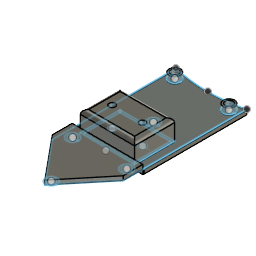
extension (Autodesk Fusion 360 design; units mm, degrees)
part number: 2025-12-24-19-58-26-619
Autodesk Fusion 360 part; units mm, degrees
sketch "Sketch1" plane through (0, 0, 0) normal (0, 0, 1) x (1, 0, 0)
  line L0 (-17.024, 124.2448) -> (-17.024, 75)
  line L1 (17.0001, 124.2453) -> (17.0001, 75)
  circle A0 centre (-13.0088, 119.745) radius 1.85
  circle A1 centre (-13.0088, 119.745) radius 2.75
  circle A2 centre (12.9912, 119.745) radius 1.85
  circle A3 centre (12.9912, 119.745) radius 2.75
  circle A4 centre (-7.3385, 84.0106) radius 1.5
  circle A5 centre (0, 96.5) radius 1.85
  circle A6 centre (0, 96.5) radius 2.75
  spline S0 degree 5 poles (-17.024, 124.2448) (-16.3297, 124.0957) (-14.9423, 123.8106) (-12.8649, 123.4218) (-10.1022, 122.9825) (-6.662, 122.574) (-3.236, 122.3191) (0.1747, 122.2305) (3.5692, 122.3158) (6.9481, 122.5687) (10.3127, 122.977) (12.9938, 123.4177) (14.9991, 123.8085) (16.3335, 124.0953) (17.0001, 124.2453) knots 0 0 0 0 0 0 0.1 0.2 0.3 0.4 0.5 0.6 0.7 0.8 0.9 1 1 1 1 1 1
  line L2 (13.0005, 74.4499) -> (-13.1768, 74.5708)
  line L3 (-13.089, 93.5708) -> (12.9107, 93.6922)
  line L4 (-13.089, 93.5708) -> (-13.1768, 74.5708)
  line L5 (13.0005, 74.4499) -> (12.9107, 93.6922)
  line L6 (-13.089, 93.5708) -> (-12.089, 93.5708) construction
  line L7 (-12.089, 93.5708) -> (-12.089, 92.5708) construction
  line L8 (-12.089, 92.5708) -> (-13.089, 92.5708) construction
  line L9 (-13.089, 92.5708) -> (-13.089, 93.5708) construction
  line L10 (13.0005, 74.4499) -> (12.0005, 74.4499) construction
  line L11 (12.0005, 74.4499) -> (12.0005, 75.4499) construction
  line L12 (12.0005, 75.4499) -> (13.0005, 75.4499) construction
  line L13 (13.0005, 75.4499) -> (13.0005, 74.4499) construction
  line L14 (-12.089, 92.5708) -> (12.0005, 92.5708)
  line L15 (12.0005, 92.5708) -> (12.0005, 75.4499)
  line L16 (12.0005, 75.4499) -> (-12.089, 75.4499)
  line L17 (-12.089, 75.4499) -> (-12.089, 92.5708)
  line L18 (-12.089, 84.0104) -> (12.0005, 84.0104) construction
  circle A7 centre (7.2615, 84.0106) radius 1.5
  circle A8 centre (0, 47.5) radius 1.85
  circle A9 centre (-13.0088, 70.745) radius 2.75
  circle A10 centre (0, 47.5) radius 2.75
  circle A11 centre (-13.0088, 70.745) radius 1.85
  line L19 (-17.024, 75) -> (-17.024, 65)
  line L20 (-17.024, 65) -> (0.0073, 44.3727)
  line L21 (0.0073, 44.3727) -> (17, 65)
  line L22 (17, 65) -> (17.0001, 75)
  circle A12 centre (12.9912, 70.745) radius 1.85
  circle A13 centre (12.9912, 70.745) radius 2.75
  point P0 (0.3284, 122.274)
  point P1 (0.3284, 73.274)
  dimension "d150" = 3.7
  dimension "d151" = 5.5
  dimension "d154" = 3.7
  dimension "d155" = 5.5
  dimension "d164" = 3
  dimension "d233" = 26.629
  dimension "d235" = 3.7
  dimension "d236" = 5.5
  dimension "d315" = 26
  dimension "d317" = 1
  dimension "d318" = 1
  dimension "d321" = 19
  dimension "d322" = 3
  dimension "d355" = 3.7
  dimension "d356" = 5.5
  dimension "d359" = 3.7
  dimension "d360" = 5.5
  dimension "d363" = 3.7
  dimension "d364" = 5.5
  constraint concentric A0 A1
  constraint concentric A2 A3
  constraint concentric A5 A6
  constraint perpendicular L2 L4
  constraint perpendicular L3 L5
  constraint horizontal L6
  constraint vertical L7
  constraint horizontal L8
  constraint vertical L9
  constraint horizontal L10
  constraint horizontal L12
  constraint horizontal L14
  constraint vertical L15
  constraint horizontal L16
  constraint vertical L17
  constraint midpoint L17 L18.start
  constraint midpoint L15 L18.end
  constraint vertical L1
  constraint vertical L0
  constraint concentric A9 A11
  constraint concentric A8 A10
  constraint parallel L0 L19
  constraint concentric A12 A13
  measures "d150" diameter of A0
  measures "d151" diameter of A1
  measures "d154" diameter of A2
  measures "d155" diameter of A3
  measures "d164" diameter of A4
  measures "d233" distance of A2.centre A5.centre
  measures "d235" diameter of A5
  measures "d236" diameter of A6
  measures "d315" distance of L3.start L3.end
  measures "d317" distance of L3.start L6.end
  measures "d318" distance of L3.start L8.end
  measures "d321" vertical distance of L3.start L2.end
  measures "d322" diameter of A7
  measures "d355" diameter of A11
  measures "d356" diameter of A9
  measures "d359" diameter of A8
  measures "d360" diameter of A10
  measures "d363" diameter of A12
  measures "d364" diameter of A13
extrude "Extrude43" add sketch "Sketch1" along normal blind 12 contours L2 L3 L4 L5 makes body 1
extrude "Extrude44" add sketch "Sketch1" along normal blind 12 contours L14 L15 L16 L17 bodies 1
extrude "Extrude45" cut sketch "Sketch1" along normal blind 8 contours L14 L15 L16 L17 bodies 1
extrude "Extrude47" add sketch "Sketch1" along normal blind 5 separate body contours A1 | A3 | A6 makes body 2 at (10.4071, 118.8045, 3.3333) makes body 3 at (-15.5929, 118.8045, 3.3333) makes body 4 at (-2.5842, 95.5594, 3.3333)
extrude "Extrude49" add sketch "Sketch1" along normal blind 2 contours L0 L1 S0 A10 L19 L20 L21 L22 | A10 L20 L21 | A10 L20 L21 | A8 | A9 | A11 | A12 | A13 bodies 1 2 3 4
fillet "Fillet6" radius 2 4 edges at (-0.0881, 74.5104, 12) (12.9556, 84.0711, 12) (-13.1329, 84.0708, 12) (-0.0892, 93.6315, 12) on bodies 1
split "Split1" by plane through (13.0005, 74.4499, 0) normal (-0.004617, -0.999989, 0) bodies 1 makes body 5 at (-0.0056, 58.1242, 0)
move_body "Move2" bodies 1 to x (1, 0, 0) y (0, 1, 0) z (0, 0, 1) at (0, 0, -2.322)
combine "Combine1" operation add target body 1 tool bodies 5
extrude "Extrude10" [suppressed]
extrude "Extrude22" [suppressed]
extrude "Extrude23" [suppressed]
extrude "Extrude24" [suppressed]
extrude "Extrude25" [suppressed]
extrude "Extrude26" [suppressed]
extrude "Extrude27" [suppressed]
delete_face "DeleteFace6" [suppressed]
extrude "Extrude28" [suppressed]
moveface "MoveFace1" [suppressed]
extrude "Extrude29" [suppressed]
extrude "Extrude30" [suppressed]
fillet "Fillet4" [suppressed]
